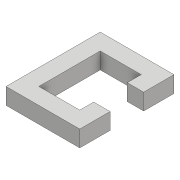
# Autodesk Inventor part: Core
Saved by Autodesk Inventor 2018.2 (Build 222227000, 227)
## iProperties
Created: 2019-02-04
Part Number: Core
Material: Generic
Document SubType Name: Modeling
Designer: ns6022
Density: 1 g/cm^3
Appearance: Default
Author: ns6022
Autodesk Inventor part; units mm, degrees
ref_plane "YZ Plane" through (0, 0, 0) normal (1, 0, 0) x (0, 1, 0)
ref_plane "XZ Plane" through (0, 0, 0) normal (0, 1, 0) x (-1, 0, 0)
ref_plane "XY Plane" through (0, 0, 0) normal (0, 0, 1) x (1, 0, 0)
sketch "Sketch1" plane through (0, 0, 0) normal (0, 0, 1) x (1, 0, 0)
  point P0 (0, 0)
sketch "LAYER1" plane through (0, 0, 0) normal (0, 0, 1) x (1, 0, 0)
  line L0 (70, 20.5) -> (90, 20.5)
  line L1 (90, 20.5) -> (90, 57.5)
  line L2 (90, 57.5) -> (0, 57.5)
  line L3 (0, 57.5) -> (0, -57.5)
  line L4 (0, -57.5) -> (90, -57.5)
  line L5 (90, -57.5) -> (90, -20.5)
  line L6 (90, -20.5) -> (70, -20.5)
  line L7 (70, -20.5) -> (70, -37.5)
  line L8 (70, -37.5) -> (20, -37.5)
  line L9 (20, -37.5) -> (20, 37.5)
  line L10 (20, 37.5) -> (70, 37.5)
  line L11 (70, 37.5) -> (70, 20.5)
  constraints: 24 end point
sketch "LAYER2" plane through (0, 0, 0) normal (0, 0, 1) x (1, 0, 0)
  line L0 (20.1, -20) -> (110.1, -20)
  line L1 (110.1, -20) -> (110.1, 20)
  line L2 (110.1, 20) -> (20.1, 20)
  line L3 (20.1, 20) -> (20.1, -20)
  constraints: 8 end point
sketch "LAYER3" plane through (0, 0, 0) normal (0, 0, 1) x (1, 0, 0)
  line L0 (20.5, -71.2) -> (69.5, -71.2)
  line L1 (69.5, -71.2) -> (69.5, -58)
  line L2 (69.5, -58) -> (20.5, -58)
  line L3 (20.5, -58) -> (20.5, -71.2)
  constraints: 8 end point
sketch "LAYER4" plane through (0, 0, 0) normal (0, 0, 1) x (1, 0, 0)
  line L0 (20.5, -23.8) -> (69.5, -23.8)
  line L1 (69.5, -23.8) -> (69.5, -37)
  line L2 (69.5, -37) -> (20.5, -37)
  line L3 (20.5, -37) -> (20.5, -23.8)
  constraints: 8 end point
sketch "LAYER5" plane through (0, 0, 0) normal (0, 0, 1) x (1, 0, 0)
  line L0 (20.5, 23.8) -> (69.5, 23.8)
  line L1 (69.5, 23.8) -> (69.5, 37)
  line L2 (69.5, 37) -> (20.5, 37)
  line L3 (20.5, 37) -> (20.5, 23.8)
  constraints: 8 end point
sketch "LAYER6" plane through (0, 0, 0) normal (0, 0, 1) x (1, 0, 0)
  line L0 (20.5, 71.2) -> (69.5, 71.2)
  line L1 (69.5, 71.2) -> (69.5, 58)
  line L2 (69.5, 58) -> (20.5, 58)
  line L3 (20.5, 58) -> (20.5, 71.2)
  constraints: 8 end point
extrude "Extrusion1" add sketch "LAYER1" along normal blind 20
body "Solid1"
